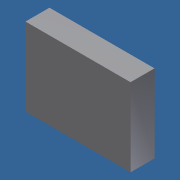
# Autodesk Inventor part: sabertooth keepout
Saved by Autodesk Inventor 2012 (Build 160160000, 160)
## iProperties
Created: 2012-03-26
Part Number: sabertooth keepout
Material: Default
Document SubType Name: Modeling
Designer: Edward
Mass: 90.7185 g
Surface Area: 180.387 cm^2
Volume: 119.298 cm^3
Density: 0.760437 g/cm^3
Author: Edward
Autodesk Inventor part; units mm, degrees
ref_plane "YZ Plane" through (0, 0, 0) normal (1, 0, 0) x (0, 1, 0)
ref_plane "XZ Plane" through (0, 0, 0) normal (0, 1, 0) x (-1, 0, 0)
ref_plane "XY Plane" through (0, 0, 0) normal (0, 0, 1) x (1, 0, 0)
sketch "Sketch1" plane through (0, 0, 0) normal (0, 0, 1) x (1, 0, 0)
  line L0 (-44.45, -33.02) -> (44.45, -33.02)
  line L1 (44.45, -33.02) -> (44.45, 33.02)
  line L2 (44.45, 33.02) -> (-44.45, 33.02)
  line L3 (-44.45, 33.02) -> (-44.45, -33.02)
  point P0 (0, 0)
  point P1 (44.45, 0)
  point P2 (0, 33.02)
  dimension "d0" = 88.9
  dimension "d1" = 66.04
  constraints: 8 end point, 2 midpoint, 2 parallel, 1 horizontal, 1 horizontal alignment, 1 perpendicular, 1 vertical alignment
  measures "d0" distance of L1.end L2.end
  measures "d1" distance between parallel lines of L2 L0
extrude "Extrusion1" add sketch "Sketch1" along normal blind 20.32
body "Solid1"
